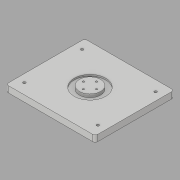
# Autodesk Inventor part: b_base_table
Saved by Autodesk Inventor 2019 (Build 230136000, 136)
## iProperties
Created: 2021-11-08
Part Number: b_base_table
Material: Generic
Document SubType Name: Modeling
Designer: Mohamed
Density: 1 g/cm^3
Appearance: Default
Author: Mohamed
Autodesk Inventor part; units mm, degrees
ref_plane "YZ Plane" through (0, 0, 0) normal (1, 0, 0) x (0, 1, 0)
ref_plane "XZ Plane" through (0, 0, 0) normal (0, 1, 0) x (-1, 0, 0)
ref_plane "XY Plane" through (0, 0, 0) normal (0, 0, 1) x (1, 0, 0)
sketch "Sketch1" plane through (0, 0, 0) normal (0, 1, 0) x (-1, 0, 0)
  line L0 (5, 0) -> (165, 0)
  line L1 (170, -5) -> (170, -145)
  line L2 (165, -150) -> (5, -150)
  line L3 (0, -145) -> (0, -5)
  arc A0 (170, -5) -> (165, 0) centre (165, -5) ccw
  arc A1 (165, -150) -> (170, -145) centre (165, -145) ccw
  arc A2 (5, 0) -> (0, -5) centre (5, -5) ccw
  arc A3 (0, -145) -> (5, -150) centre (5, -145) ccw
  point P0 (0, 0)
  point P1 (170, -150)
  point P2 (170, 0)
  point P3 (0, -150)
  dimension "d0" = 170
  dimension "d1" = 150
  dimension "d2" = 5
  constraints: 8 end point, 8 point on circle, 8 point on line, 8 tangent, 4 centre point, 3 equal radius, 2 parallel, 1 horizontal, 1 perpendicular
  measures "d0" distance of point (170, -150) point (0, -150)
  measures "d1" distance of point (170, 0) point (170, -150)
  measures "d2" radius of A0
extrude "Extrusion1" add sketch "Sketch1" along normal blind 12
sketch "Sketch2" plane through (0, 12, 0) normal (0, 1, 0) x (1, 0, 0)
  line L0 (0, 5) -> (0, 145) projected
  line L1 (-170, 145) -> (-170, 5) projected
  line L2 (-165, 0) -> (-5, 0) projected
  circle A0 centre (-85, 75) radius 20
  circle A1 centre (-85, 75) radius 30
  point P0 (0, 0)
  dimension "d5" = 40
  dimension "d6" = 60
  constraints: 2 centre point, 1 coincident
  measures "d5" diameter of A0
  measures "d6" diameter of A1
extrude "Extrusion2" cut sketch "Sketch2" against normal blind 3
sketch "Sketch3" plane through (-85, 12, -75) normal (0, 1, 0) x (1, 0, 0)
  circle A0 centre (0, 0) radius 30 projected
  circle A1 centre (0, 0) radius 20
  point P0 (85, -75)
  constraints: 1 centre point, 1 coincident
extrude "Extrusion3" add sketch "Sketch3" along normal blind 3 contours A1
sketch "Sketch4" plane through (-85, 15, -75) normal (0, 1, 0) x (1, 0, 0)
  circle A0 centre (-12.5, 0) radius 1.75
  circle A1 centre (0, 12.5) radius 1.75
  circle A2 centre (0, -12.5) radius 1.75
  circle A3 centre (12.5, 0) radius 1.75
  point P0 (85, -75)
  dimension "d15" = 3.5
  dimension "d16" = 3.5
  dimension "d17" = 3.5
  dimension "d18" = 3.5
  constraints: 4 centre point
  measures "d15" diameter of A0
  measures "d16" diameter of A1
  measures "d17" diameter of A2
  measures "d18" diameter of A3
extrude "Extrusion4" cut sketch "Sketch4" against normal blind 20
sketch "Sketch5" plane through (0, 0, 0) normal (0, -1, 0) x (1, 0, 0)
  circle A0 centre (-85, -87.5) radius 1.75 projected
  circle A1 centre (-85, -87.5) radius 3.5
  circle A2 centre (-72.5, -75) radius 1.75 projected
  circle A3 centre (-72.5, -75) radius 3.5
  circle A4 centre (-85, -62.5) radius 1.75 projected
  circle A5 centre (-85, -62.5) radius 3.5
  circle A6 centre (-97.5, -75) radius 1.75 projected
  circle A7 centre (-97.5, -75) radius 3.5
  point P0 (0, 0)
  dimension "d21" = 7
  dimension "d22" = 7
  dimension "d23" = 7
  dimension "d24" = 7
  constraints: 4 centre point, 4 coincident
  measures "d21" diameter of A1
  measures "d22" diameter of A3
  measures "d23" diameter of A5
  measures "d24" diameter of A7
extrude "Extrusion5" cut sketch "Sketch5" against normal blind 4
sketch "Sketch6" plane through (0, 0, 0) normal (0, -1, 0) x (1, 0, 0)
  line L0 (0, 0) -> (0, -20)
  line L1 (0, -5) -> (0, -145) projected
  line L2 (0, -20) -> (-15, -20)
  line L3 (0, -150) -> (0, -130)
  line L4 (0, -130) -> (-15, -130)
  line L5 (-170, 0) -> (-170, -20)
  line L6 (-170, -145) -> (-170, -5) projected
  line L7 (-170, -20) -> (-155, -20)
  line L8 (-170, -150) -> (-170, -130)
  line L9 (-170, -130) -> (-155, -130)
  circle A0 centre (-15, -20) radius 2.45
  circle A1 centre (-15, -130) radius 2.45
  circle A2 centre (-155, -20) radius 2.45
  circle A3 centre (-155, -130) radius 2.45
  dimension "d27" = 20
  dimension "d28" = 15
  dimension "d29" = 20
  dimension "d30" = 15
  dimension "d31" = 20
  dimension "d32" = 15
  dimension "d33" = 20
  dimension "d34" = 15
  dimension "d35" = 4.9
  dimension "d36" = 4.9
  dimension "d37" = 4.9
  dimension "d38" = 4.9
  constraints: 16 end point, 4 centre point, 4 coincident, 4 perpendicular, 4 point on line
  measures "d27" distance of L0.start L0.end
  measures "d28" distance of L0.end L2.end
  measures "d29" distance of L3.start L3.end
  measures "d30" distance of L3.end L4.end
  measures "d31" distance of L5.start L5.end
  measures "d32" distance of L5.end L7.end
  measures "d33" distance of L8.start L8.end
  measures "d34" distance of L8.end L9.end
  measures "d35" diameter of A0
  measures "d36" diameter of A1
  measures "d37" diameter of A2
  measures "d38" diameter of A3
extrude "Extrusion6" cut sketch "Sketch6" against normal blind 15
body "Solid1"
